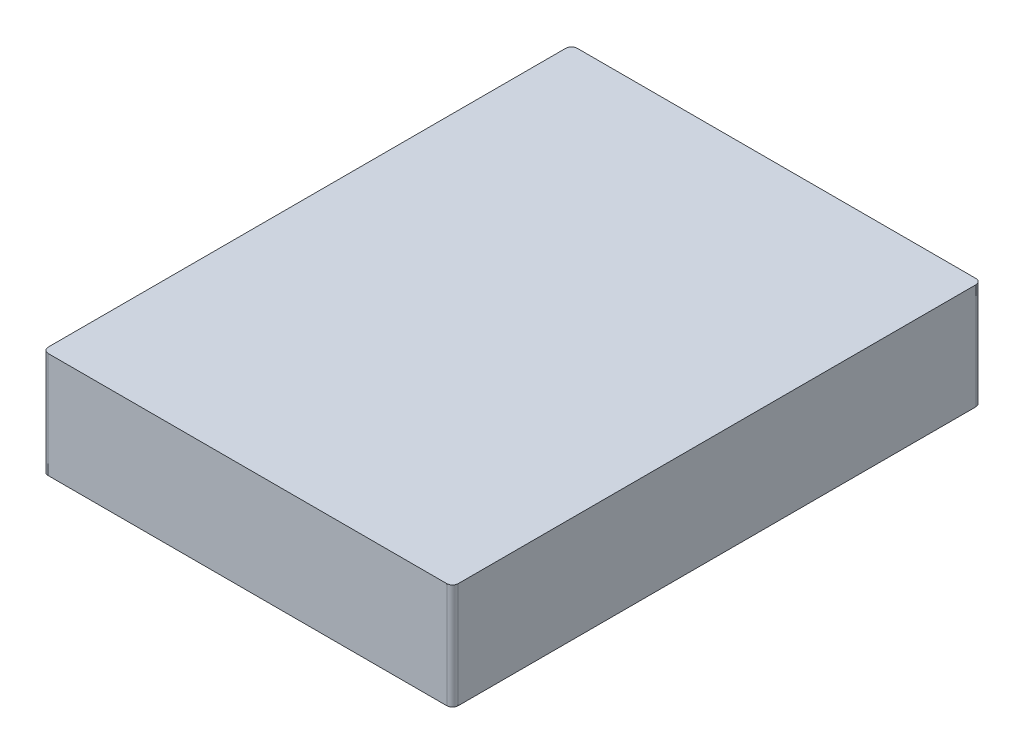
# Autodesk Inventor part: esc
Saved by Autodesk Inventor 2021 (Build 250183000, 183)
## iProperties
Created: 2021-01-20
Part Number: esc
Material: ABS Plastic
Document SubType Name: Modeling
Designer: User
Density: 1.06 g/cm^3
Appearance: Smooth - Black
Author: User
Autodesk Inventor part; units mm, degrees
ref_plane "YZ Plane" through (0, 0, 0) normal (1, 0, 0) x (0, 1, 0)
ref_plane "XZ Plane" through (0, 0, 0) normal (0, 1, 0) x (-1, 0, 0)
ref_plane "XY Plane" through (0, 0, 0) normal (0, 0, 1) x (1, 0, 0)
sketch "Sketch18" plane through (0, 0, 0) normal (0, 1, 0) x (-1, 0, 0)
  line L0 (15.5, 20) -> (-15.5, 20)
  line L1 (-15.5, 20) -> (-15.5, -20)
  line L2 (-15.5, -20) -> (15.5, -20)
  line L3 (15.5, -20) -> (15.5, 20)
  line L4 (15.5, 20) -> (-15.5, -20) construction
  line L5 (-15.5, 20) -> (15.5, -20) construction
  point P0 (0, 0)
  dimension "d163" = 31
  dimension "d164" = 40
  constraints: 12 end point, 2 midpoint, 2 parallel, 1 horizontal, 1 perpendicular
  measures "d163" distance of L2.end L1.end
  measures "d164" distance of L1.end L0.end
extrude "Extrusion17" add sketch "Sketch18" along normal blind 8
fillet "Fillet7" radius 0.4 4 edges at (15.5, 4, 20) (-15.5, 4, 20) (-15.5, 4, -20) (15.5, 4, -20)
body "Solid4"
